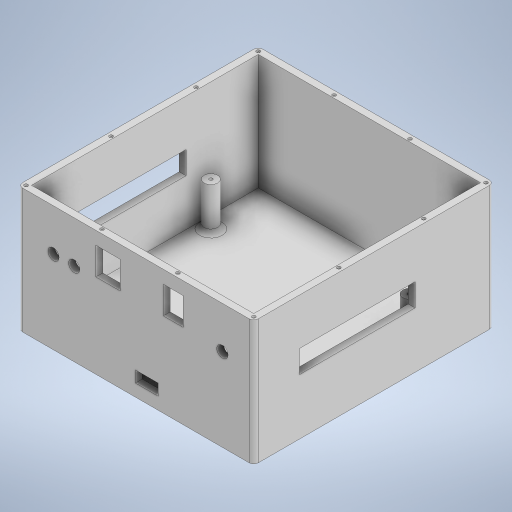
# Autodesk Inventor part: Base Chassis
Saved by Autodesk Inventor 2023 (Build 270158000, 158)
## iProperties
Created: 2023-03-17
Part Number: Base Chassis
Material: Generic
Document SubType Name: Modeling
Designer: Ahmed Nazir
Density: 1 g/cm^3
Appearance: Default
Author: Ahmed Nazir
Autodesk Inventor part; units mm, degrees
ref_plane "YZ Plane" through (0, 0, 0) normal (1, 0, 0) x (0, 1, 0)
ref_plane "XZ Plane" through (0, 0, 0) normal (0, 1, 0) x (-1, 0, 0)
ref_plane "XY Plane" through (0, 0, 0) normal (0, 0, 1) x (1, 0, 0)
sketch "Sketch1" plane through (0, 0, 0) normal (0, 1, 0) x (-1, 0, 0)
  line L0 (0, 0) -> (-98, 0)
  line L1 (-98, 0) -> (-98, -100)
  line L2 (-98, -100) -> (0, -100)
  line L3 (0, -100) -> (0, 0)
  line L4 (3, -103) -> (-101, -103)
  line L5 (-101, -103) -> (-101, 3)
  line L6 (-101, 3) -> (3, 3)
  line L7 (3, 3) -> (3, -103)
  line L8 (0, -20) -> (-6, -20)
  line L9 (-6, -20) -> (-6, -80)
  line L10 (-6, -80) -> (0, -80)
  line L11 (0, -80) -> (0, -20)
  line L12 (-46, -20) -> (-52, -20)
  line L13 (-52, -20) -> (-52, -80)
  line L14 (-52, -80) -> (-46, -80)
  line L15 (-46, -80) -> (-46, -20)
  line L16 (-92, -20) -> (-98, -20)
  line L17 (-98, -20) -> (-98, -80)
  line L18 (-98, -80) -> (-92, -80)
  line L19 (-92, -80) -> (-92, -20)
  point P0 (-49, -20)
  point P1 (-6, -50)
  point P2 (-98, -20)
  point P3 (-98, -80)
  point P4 (0, -80)
  point P5 (0, -20)
  dimension "d0" = 100
  dimension "d1" = 98
  dimension "d2" = 3
  dimension "d48" = 6
  dimension "d49" = 60
  dimension "d50" = 6
  dimension "d51" = 60
  dimension "d52" = 6
  dimension "d53" = 60
  dimension "d54" = 49
  dimension "d55" = 50
  constraints: 40 end point, 10 parallel, 5 perpendicular, 4 horizontal, 2 collinear, 2 midpoint, 2 point on line, 3 other
  measures "d0" distance of L1.end L0.end
  measures "d1" distance of L1.end L2.end
  measures "d2" distance between parallel lines of L2 L4
  measures "d48" distance of L10.end L9.end
  measures "d49" distance of L9.end L8.end
  measures "d50" distance of L14.end L13.end
  measures "d51" distance of L13.end L12.end
  measures "d52" distance of L18.end L17.end
  measures "d53" distance of L17.end L16.end
  measures "d54" distance from line of L1 point (-49, -20)
  measures "d55" distance from line of L0 point (-6, -50)
extrude "Extrusion1" add sketch "Sketch1" along normal blind 4 contours L3 L8 L9 L10 L2 L1 L18 L19 L16 L0 | L3 L10 L9 L8 | L16 L19 L18 L1 | L15 L14 L13 L12
extrude "Extrusion2" add sketch "Sketch1" along normal blind 55 contours L4 L5 L6 L7
fillet "Fillet1" radius 2 4 edges at (-3, 27.5, 3) (101, 27.5, 3) (101, 27.5, -103) (-3, 27.5, -103)
sketch "Sketch2" plane through (0, 4, 0) normal (0, 1, 0) x (1, 0, 0)
  line L0 (98, 0) -> (98, 100) projected
  line L1 (98, 100) -> (0, 100) projected
  line L2 (0, 100) -> (0, 0) projected
  line L3 (0, 0) -> (98, 0) projected
  circle A0 centre (5.185, 73.913) radius 3
  circle A1 centre (5.185, 6.858) radius 3
  circle A2 centre (92.815, 6.858) radius 3
  circle A3 centre (92.815, 73.913) radius 3
  dimension "d8" = 6
  dimension "d9" = 6
  dimension "d10" = 6
  dimension "d11" = 6
  dimension "d12" = 67.055
  dimension "d13" = 87.63
  dimension "d16" = 6.858
  dimension "d17" = 5.185
  constraints: 4 centre point, 2 horizontal alignment, 2 vertical alignment
  measures "d8" diameter of A0
  measures "d9" diameter of A1
  measures "d10" diameter of A2
  measures "d11" diameter of A3
  measures "d12" distance of A1.centre A0.centre
  measures "d13" distance of A3.centre A0.centre
  measures "d16" distance from line of L3 A1.centre
  measures "d17" distance from line of L2 A1.centre
extrude "Extrusion3" add sketch "Sketch2" along normal blind 19 contours A0 | A1 | A2 | A3
sketch "Sketch3" plane through (92.815, 23, -73.913) normal (0, 1, 0) x (1, 0, 0)
  circle A0 centre (0, -67.055) radius 3 projected
  circle A1 centre (0, -67.055) radius 0.75
  circle A2 centre (0, 0) radius 3 projected
  circle A3 centre (0, 0) radius 0.75
  circle A4 centre (-87.63, 0) radius 3 projected
  circle A5 centre (-87.63, 0) radius 0.75
  circle A6 centre (-87.63, -67.055) radius 3 projected
  circle A7 centre (-87.63, -67.055) radius 0.75
  point P0 (-92.815, -73.913)
  dimension "d21" = 1.5
  dimension "d22" = 1.5
  dimension "d23" = 1.5
  dimension "d24" = 1.5
  constraints: 4 centre point, 4 coincident
  measures "d21" diameter of A1
  measures "d22" diameter of A3
  measures "d23" diameter of A5
  measures "d24" diameter of A7
extrude "Extrusion4" cut sketch "Sketch3" against normal blind 5 contours A1 | A3 | A5 | A7
fillet "Fillet2" radius 2 4 edges at (89.815, 4, -73.913) (89.815, 4, -6.858) (2.185, 4, -6.858) (2.185, 4, -73.913)
extrude "Extrusion5" cut sketch "Sketch1" along normal blind 2 contours L3 L10 L9 L8 | L16 L19 L18 L1 | L15 L14 L13 L12
sketch "Sketch4" plane through (-1, 0, 3) normal (0, 0, 1) x (1, 0, 0)
  line L0 (11.185, 4) -> (1.185, 4) projected
  line L1 (98.815, 4) -> (88.815, 4) projected
  line L2 (99, 4) -> (1, 4) projected
  line L3 (1, 4) -> (99, 4) projected
  line L4 (98.815, 4) -> (88.815, 4) projected
  line L5 (11.185, 4) -> (1.185, 4) projected
  line L6 (1, 4) -> (1, 55) projected
  line L7 (1, 4) -> (1, 55) projected
  line L8 (99, 4) -> (99, 55) projected
  line L9 (99, 4) -> (99, 55) projected
  line L10 (43.14, 49.31) -> (32.39, 49.31)
  line L11 (32.39, 49.31) -> (32.39, 37.21)
  line L12 (32.39, 37.21) -> (43.14, 37.21)
  line L13 (43.14, 37.21) -> (43.14, 49.31)
  line L14 (49.815, 5.39) -> (59.815, 5.39)
  line L15 (59.815, 5.39) -> (59.815, 10.39)
  line L16 (59.815, 10.39) -> (49.815, 10.39)
  line L17 (49.815, 10.39) -> (49.815, 5.39)
  line L18 (62.14, 49.31) -> (70.89, 49.31)
  line L19 (70.89, 49.31) -> (70.89, 37.21)
  line L20 (70.89, 37.21) -> (62.14, 37.21)
  line L21 (62.14, 37.21) -> (62.14, 49.31)
  line L22 (9.185, 23) -> (3.185, 23) projected
  line L23 (96.815, 23) -> (90.815, 23) projected
  circle A0 centre (13.6833, 36.5386) radius 2.5
  circle A1 centre (22.8325, 36.5386) radius 2.5
  circle A2 centre (88.2047, 36.5386) radius 2.5
  point P0 (1, 0)
  point P1 (66.515, 37.21)
  point P2 (70.89, 43.26)
  point P3 (59.815, 7.89)
  point P4 (49.815, 7.89)
  point P5 (54.815, 5.39)
  point P6 (54.815, 10.39)
  point P7 (6.185, 23)
  point P8 (37.765, 37.21)
  point P9 (93.815, 23)
  dimension "d56" = 12.1
  dimension "d57" = 19
  dimension "d59" = 10.75
  dimension "d60" = 12.1
  dimension "d61" = 8.75
  dimension "d62" = 10
  dimension "d63" = 5
  dimension "d103" = 12.61
  dimension "d105" = 14.21
  dimension "d106" = 39
  dimension "d107" = 27.3
  dimension "d108" = 5
  dimension "d109" = 5
  dimension "d110" = 5
  constraints: 24 end point, 9 midpoint, 6 parallel, 3 centre point, 3 horizontal, 3 perpendicular, 2 horizontal alignment, 1 collinear
  measures "d56" distance between parallel lines of L12 L10
  measures "d57" distance between parallel lines of L21 L13
  measures "d59" distance of L10.start L10.end
  measures "d60" distance from line of point (66.515, 37.21) L18
  measures "d61" distance from line of point (70.89, 43.26) L21
  measures "d62" distance of point (59.815, 7.89) point (49.815, 7.89)
  measures "d63" distance of point (54.815, 5.39) point (54.815, 10.39)
  measures "d103" distance between parallel lines of L16 L22
  measures "d105" vertical distance of point (6.185, 23) point (37.765, 37.21)
  measures "d106" horizontal distance of point (93.815, 23) point (54.815, 10.39)
  measures "d107" horizontal distance of point (93.815, 23) point (66.515, 37.21)
  measures "d108" diameter of A0
  measures "d109" diameter of A1
  measures "d110" diameter of A2
extrude "Extrusion6" cut sketch "Sketch4" against normal up to surface (3 mm away)
sketch "Sketch5" plane through (101, 0, 1) normal (1, 0, 0) x (0, 0, -1)
  line L0 (12.858, 4) -> (2.858, 4) projected
  line L1 (79.913, 4) -> (69.913, 4) projected
  line L2 (1, 4) -> (101, 4) projected
  line L3 (101, 4) -> (1, 4) projected
  line L4 (12.858, 4) -> (2.858, 4) projected
  line L5 (79.913, 4) -> (69.913, 4) projected
  line L6 (1, 37.21) -> (1, 49.31) projected
  line L7 (1, 49.31) -> (1, 37.21) projected
  line L8 (1, 49.31) -> (1, 37.21) projected
  line L9 (1, 37.21) -> (1, 49.31) projected
  line L10 (1, 4) -> (1, 55) projected
  line L11 (1, 4) -> (1, 55) projected
  line L12 (10.858, 23) -> (4.858, 23) projected
  line L13 (77.913, 23) -> (71.913, 23) projected
  line L14 (18.133, 24.6) -> (69.133, 24.6)
  line L15 (69.133, 24.6) -> (69.133, 34.6)
  line L16 (69.133, 34.6) -> (18.133, 34.6)
  line L17 (18.133, 34.6) -> (18.133, 24.6)
  line L18 (12.858, 4) -> (2.858, 4) projected
  line L19 (4.858, 6) -> (10.858, 6) projected
  line L20 (79.913, 4) -> (69.913, 4) projected
  line L21 (71.913, 6) -> (77.913, 6) projected
  line L22 (1, 10.39) -> (1, 5.39) projected
  line L23 (1, 5.39) -> (1, 10.39) projected
  point P0 (1, 0)
  point P1 (74.913, 23)
  dimension "d98" = 10
  dimension "d99" = 51
  dimension "d101" = 1.6
  dimension "d102" = 5.78
  constraints: 8 end point, 2 parallel, 1 horizontal, 1 midpoint, 1 perpendicular
  measures "d98" distance between parallel lines of L14 L16
  measures "d99" distance of L15.end L16.end
  measures "d101" distance between parallel lines of L13 L14
  measures "d102" distance from line of point (74.913, 23) L15
sketch "Sketch6" plane through (-3, 0, -101) normal (-1, 0, 0) x (0, 0, 1)
  line L0 (32.867, 34.6) -> (83.867, 34.6) projected
  line L1 (32.867, 24.6) -> (32.867, 34.6) projected
  line L2 (83.867, 24.6) -> (32.867, 24.6) projected
  line L3 (83.867, 34.6) -> (83.867, 24.6) projected
  point P0 (101, 0)
extrude "Extrusion7" cut sketch "Sketch5" against normal up to surface (3 mm away)
extrude "Extrusion8" cut sketch "Sketch6" against normal up to surface (3 mm away)
sketch "Sketch7" plane through (0, 55, 0) normal (0, 1, 0) x (1, 0, 0)
  circle A0 centre (-1.2, -1.2) radius 0.8
  circle A1 centre (99.2, -1.2) radius 0.8
  line L0 (98, 100) -> (98, 0) projected
  circle A2 centre (99.2, 101.2) radius 0.8
  line L1 (0, 100) -> (98, 100) projected
  circle A3 centre (-1.2, 101.2) radius 0.8
  line L2 (0, 0) -> (0, 100) projected
  circle A4 centre (32.27, -1.2) radius 0.8
  circle A5 centre (32.27, 101.2) radius 0.8
  circle A6 centre (65.74, -1.2) radius 0.8
  circle A7 centre (65.74, 101.2) radius 0.8
  circle A8 centre (-1.2, 36.27) radius 0.8
  circle A9 centre (99.2, 36.27) radius 0.8
  circle A10 centre (-1.2, 73.74) radius 0.8
  circle A11 centre (99.2, 73.74) radius 0.8
  dimension "d1" = 98
  dimension "d64" = 1.6
  dimension "d65" = 1.2
  dimension "d66" = 1.2
  dimension "d67" = 1.6
  dimension "d68" = 1.2
  dimension "d69" = 1.6
  dimension "d70" = 1.2
  dimension "d71" = 1.2
  dimension "d72" = 1.6
  dimension "d73" = 1.2
  dimension "d74" = 1.2
  dimension "d87" = 33.47
  dimension "d91" = 37.47
  constraints: 12 centre point, 1 horizontal, 1 horizontal alignment, 1 vertical, 16 other
  measures "d64" diameter of A0
  measures "d65" horizontal distance of A0.centre L2.start
  measures "d66" horizontal distance of L2.start A0.centre
  measures "d67" diameter of A1
  measures "d68" distance from line of L0 A1.centre
  measures "d69" diameter of A2
  measures "d70" distance from line of L0 A2.centre
  measures "d71" distance from line of A2.centre L1
  measures "d72" diameter of A3
  measures "d73" distance from line of A3.centre L1
  measures "d74" distance from line of L2 A3.centre
  measures "d87" distance of A0.centre A4.centre
  measures "d91" distance of A0.centre A8.centre
extrude "Extrusion9" cut sketch "Sketch7" against normal blind 0.8
equation "\"d54\" = 0.5 * d1"
equation "\"d55\" = 0.5 * d0"
equation "\"d60\" = d56"
body "Solid1"
